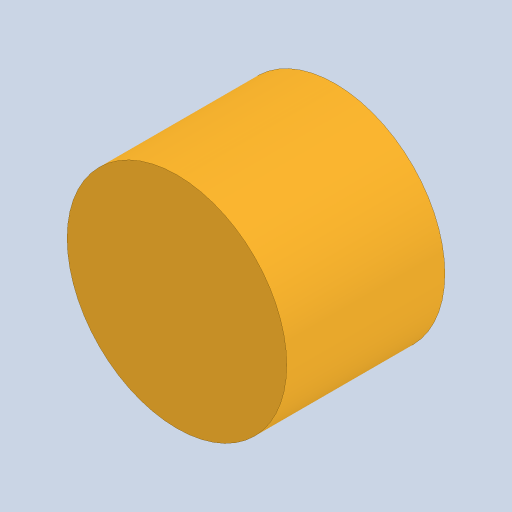
# Autodesk Inventor part: Heis_kopp
Saved by Autodesk Inventor 2023.1 (Build 271208000, 208)
## iProperties
Created: 2024-07-19
Part Number: Heis_kopp
Material: S355J2+N
Document SubType Name: Modeling
Designer: huchonms
Engineer: thingelstade
Mass: 45.5675 g
Surface Area: 26.7467 cm^2
Volume: 5.80477 cm^3
Density: 7.85 g/cm^3
Appearance: Metal (300-500 MPa)
tc_part_rev_length: 25
tc_part_rev_width: 18
tc_part_rev_height: 25
tc_part_rev_uom_length: mm
tc_part_rev_volume: 5805
tc_part_rev_uom_volume: mm^3
tc_part_rev_mass: 0.05
tc_part_rev_uom_mass: kg
NOV_FileName: Heis_kopp
Author: huchonms
Revision Number: 0
Autodesk Inventor part; units mm, degrees
ref_plane "YZ Plane" through (0, 0, 0) normal (1, 0, 0) x (0, 1, 0)
ref_plane "XZ Plane" through (0, 0, 0) normal (0, 1, 0) x (-1, 0, 0)
ref_plane "XY Plane" through (0, 0, 0) normal (0, 0, 1) x (1, 0, 0)
sketch "Sketch1" plane through (0, 0, 0) normal (0, 1, 0) x (-1, 0, 0)
  circle A0 centre (0, 0) radius 12.5
  dimension "d0" = 25
  constraints: 1 centre point, 1 coincident
  measures "d0" diameter of A0
extrude "Extrusion1" add sketch "Sketch1" along normal blind 2.5
sketch "Sketch2" plane through (0, 2.5, 0) normal (0, 1, 0) x (1, 0, 0)
  circle A0 centre (0, 0) radius 11.5
  dimension "d3" = 23
  constraints: 1 centre point, 1 coincident
  measures "d3" diameter of A0
extrude "Extrusion2" cut sketch "Sketch2" against normal blind 1
sketch "Sketch3" plane through (0, 2.5, 0) normal (0, 1, 0) x (1, 0, 0)
  circle A0 centre (0, 0) radius 11.5 projected
  circle A1 centre (0, 0) radius 12.5 projected
  line L0 (-8.2614, -8) -> (-9.6047, -8)
  line L1 (-8.2614, 8) -> (-9.6047, 8)
  constraints: 4 end point, 4 point on circle, 1 horizontal, 1 parallel
extrude "Extrusion3" cut sketch "Sketch3" against normal up to surface (1 mm away) contours A0 L0 A1 L1 picked at (-11.7871, 0)
sketch "Sketch6" plane through (0, 2.5, 0) normal (0, 1, 0) x (1, 0, 0)
  arc A0 (-9.6047, -8) -> (-9.6047, 8) centre (0, 0) ccw projected
  arc A1 (-8.2614, -8) -> (-8.2614, 8) centre (0, 0) ccw projected
  line L0 (-9.6047, 8) -> (-8.2614, 8) projected
  line L1 (-8.2614, -8) -> (-9.6047, -8) projected
extrude "Extrusion5" add sketch "Sketch6" along normal blind 1
sketch "Sketch7" plane through (0, 3.5, 0) normal (0, 1, 0) x (1, 0, 0)
  arc A0 (-8.2614, -8) -> (-8.2614, 8) centre (0, 0) ccw projected
  line L0 (-9.6047, 8) -> (-8.2614, 8) projected
  line L1 (-8.2614, -8) -> (-9.6047, -8) projected
  arc A1 (-9.6047, -8) -> (-9.6047, 8) centre (0, 0) ccw projected
extrude "Extrusion6" add sketch "Sketch7" along normal blind 5
sketch "Sketch8" plane through (0, 0, 0) normal (0, -1, 0) x (1, 0, 0)
  circle A0 centre (0, 0) radius 12.5 projected
extrude "Extrusion7" add sketch "Sketch8" along normal blind 4.5
sketch "Sketch9" plane through (0, -4.5, 0) normal (0, -1, 0) x (1, 0, 0)
  circle A0 centre (0, 0) radius 12.5 projected
extrude "Extrusion8" add sketch "Sketch9" along normal blind 5
body "Solid1"
